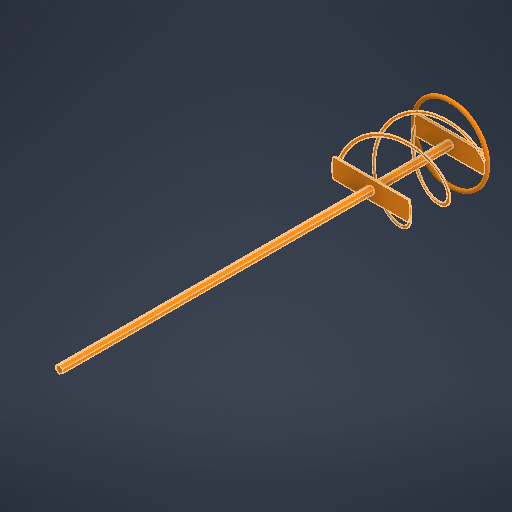
# Autodesk Inventor part: MEZCLADOR-TRUPPER-80MM
Saved by Autodesk Inventor 2025.3 (Build 293356030, 356C)
## iProperties
Created: 2025-10-05
Part Number: MEZCLADOR-TRUPPER-80MM
Material: Generic
Document SubType Name: Modeling
Designer: lstk1ng
Density: 1 g/cm^3
Appearance: Orange
Author: lstk1ng
Autodesk Inventor part; units mm, degrees
ref_plane "YZ Plane" through (0, 0, 0) normal (1, 0, 0) x (0, 1, 0)
ref_plane "XZ Plane" through (0, 0, 0) normal (0, 1, 0) x (-1, 0, 0)
ref_plane "XY Plane" through (0, 0, 0) normal (0, 0, 1) x (1, 0, 0)
sketch "Sketch1" plane through (0, 0, 0) normal (0, 1, 0) x (-1, 0, 0)
  line L0 (0, 0) -> (-40, 0) construction
  line L1 (-40, 0) -> (-38, 0) construction
  circle A0 centre (-38, 0) radius 2
  line L2 (0, -2.8) -> (0, 2.8) projected
  dimension "d0" = 40
  dimension "d1" = 2
  constraints: 4 end point, 1 coincident, 1 horizontal, 1 horizontal alignment, 1 point on line, 2 other
  measures "d0" distance of L0.start L0.end
  measures "d1" distance of L0.end L1.end
revolve "Revolution1" add sketch "Sketch1" angle 360 about axis through (0, 0, -10) along (0, 0, 1)
sketch "Sketch2" plane through (0, 0, 0) normal (0, 0, 1) x (1, 0, 0)
  line L0 (-36, 10) -> (36, 10)
  line L1 (-36, -10) -> (36, -10)
  line L2 (-36, 10) -> (-37, 10)
  line L3 (-37, 10) -> (-37, -10)
  line L4 (-37, -10) -> (-36, -10)
  line L5 (36, 10) -> (37, 10)
  line L6 (37, 10) -> (37, -10)
  line L7 (37, -10) -> (36, -10)
  point P0 (0, 0)
  point P1 (0, 0)
  dimension "d5" = 1
  dimension "d6" = 1
  constraints: 16 end point, 4 perpendicular, 2 horizontal
  measures "d5" distance of L0.start L2.end
  measures "d6" distance of L0.end L5.end
extrude "Extrusion1" add sketch "Sketch2" along normal mid plane 2
ref_plane "Work Plane1" through (0, 0, 81) normal (0, 0, 1) x (1, 0, 0)
sketch "Sketch3" plane through (0, 0, 81) normal (0, 0, 1) x (1, 0, 0)
  circle A0 centre (0, 0) radius 40 projected
  line L0 (-38.7298, -10) -> (38.7298, -10)
  line L1 (-38.7298, 10) -> (38.7298, 10)
  constraints: 4 end point, 4 point on circle, 2 horizontal
extrude "Extrusion2" add sketch "Sketch3" along normal mid plane 1.5 contours A0 L0 L1
sketch "Sketch4" plane through (0, 0, 80.25) normal (0, 0, -1) x (-1, 0, 0)
  line L0 (34.768, 1) -> (37.768, 1)
  line L1 (37.768, 1) -> (37.768, -1)
  line L2 (37.768, -1) -> (34.768, -1)
  line L3 (34.768, -1) -> (34.768, 1)
  line L4 (34.768, 1) -> (37.768, -1) construction
  line L5 (37.768, 1) -> (34.768, -1) construction
  line L6 (-37.518, 0.75) -> (-35.018, 0.75)
  line L7 (-35.018, 0.75) -> (-35.018, -0.75)
  line L8 (-35.018, -0.75) -> (-37.518, -0.75)
  line L9 (-37.518, -0.75) -> (-37.518, 0.75)
  line L10 (-37.518, 0.75) -> (-35.018, -0.75) construction
  line L11 (-35.018, 0.75) -> (-37.518, -0.75) construction
  point P0 (0, 0)
  point P1 (36.268, 0)
  point P2 (-36.268, 0)
  dimension "d18" = 3
  dimension "d19" = 2
  dimension "d20" = 2.5
  dimension "d21" = 1.5
  constraints: 24 end point, 4 midpoint, 4 parallel, 2 horizontal, 2 perpendicular
  measures "d18" distance of L1.end L2.end
  measures "d19" distance of L0.end L1.end
  measures "d20" distance of L7.end L8.end
  measures "d21" distance of L6.end L7.end
sketch3d "3D Sketch1"
  helix H0 starts at (-36.268, 0, 0) axis through (0, 0, 0) along (0, 0, 1) pitch 80 turns 1 hand right
sweep "Sweep1" add profiles "Sketch4" path "3D Sketch1"
sketch "Sketch5" plane through (0, 0, 1) normal (0, 0, 1) x (1, 0, 0)
  line L0 (0, 3.9) -> (3.3775, 1.95)
  line L1 (3.3775, 1.95) -> (3.3775, -1.95)
  line L2 (3.3775, -1.95) -> (0, -3.9)
  line L3 (0, -3.9) -> (-3.3775, -1.95)
  line L4 (-3.3775, -1.95) -> (-3.3775, 1.95)
  line L5 (-3.3775, 1.95) -> (0, 3.9)
  point P0 (0, 0)
  point P1 (0, 0)
  dimension "d32" = 7.8
  constraints: 12 end point, 1 coincident, 13 other
  measures "d32" distance of L2.end L0.start
extrude "Extrusion3" add sketch "Sketch5" along normal blind 400
body "Solid1"
